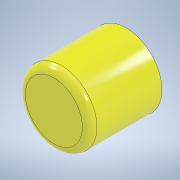
# Autodesk Inventor part: Mini Lights Yellow
Saved by Autodesk Inventor 2022.1 (Build 261234000, 234)
## iProperties
Created: 2023-05-17
Part Number: Mini Lights Yellow
Material: Generic
Document SubType Name: Modeling
Designer: brenden_deutschman
Density: 1 g/cm^3
Appearance: Default
Author: brenden_deutschman
Autodesk Inventor part; units mm, degrees
ref_plane "YZ Plane" through (0, 0, 0) normal (1, 0, 0) x (0, 1, 0)
ref_plane "XZ Plane" through (0, 0, 0) normal (0, 1, 0) x (-1, 0, 0)
ref_plane "XY Plane" through (0, 0, 0) normal (0, 0, 1) x (1, 0, 0)
sketch "Sketch1" plane through (0, 0, 0) normal (0, 0, 1) x (1, 0, 0)
  circle A0 centre (0, 0) radius 2.5
  dimension "d0" = 5
  constraints: 1 centre point, 1 coincident
  measures "d0" diameter of A0
extrude "Extrusion1" add sketch "Sketch1" against normal blind 5.0457
fillet "Face Fillet1" radius 0.508 1 edges at (-2.5, 0, 0)
body "Solid1"
